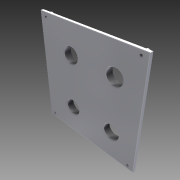
# Autodesk Inventor part: SinglePlane3
Saved by Autodesk Inventor 2015 (Build 190159000, 159)
## iProperties
Created: 2015-03-20
Part Number: SinglePlane3
Material: Aluminum 6061
Document SubType Name: Modeling
Designer: Akovo_000
Density: 2.7 g/cm^3
Appearance: Aluminum - Flat
Mass: 35.5834 g
Surface Area: 130.658 cm^2
Volume: 13.1791 cm^3
Author: Akovo_000
Autodesk Inventor part; units mm, degrees
ref_plane "YZ Plane" through (0, 0, 0) normal (1, 0, 0) x (0, 1, 0)
ref_plane "XZ Plane" through (0, 0, 0) normal (0, 1, 0) x (-1, 0, 0)
ref_plane "XY Plane" through (0, 0, 0) normal (0, 0, 1) x (1, 0, 0)
ref_plane "Main Work Pane" through (0, 2.75, 7) normal (0, 1, 0) x (-1, 0, 0)
sketch "Panel" plane through (0, 2.75, 7) normal (0, 1, 0) x (-1, 0, 0)
  circle A0 centre (8.8252, 26.2409) radius 5.8
  circle A1 centre (8.8252, -12.7591) radius 5.8
  circle A2 centre (42.6252, -12.7591) radius 5.8
  circle A3 centre (42.6252, 26.2409) radius 5.8
  line L0 (42.6252, -12.7591) -> (42.6252, -12.7591)
  line L1 (60.6252, 44.2409) -> (24.6252, 44.2409)
  line L2 (24.6252, 44.2409) -> (24.6252, 8.2409)
  line L3 (24.6252, 8.2409) -> (60.6252, 8.2409)
  line L4 (60.6252, 8.2409) -> (60.6252, 44.2409)
  line L5 (60.6252, 44.2409) -> (24.6252, 8.2409) construction
  line L6 (24.6252, 44.2409) -> (60.6252, 8.2409) construction
  line L7 (60.6252, 5.2409) -> (24.6252, 5.2409)
  line L8 (24.6252, 5.2409) -> (24.6252, -30.7591)
  line L9 (24.6252, -30.7591) -> (60.6252, -30.7591)
  line L10 (60.6252, -30.7591) -> (60.6252, 5.2409)
  line L11 (60.6252, 5.2409) -> (24.6252, -30.7591) construction
  line L12 (24.6252, 5.2409) -> (60.6252, -30.7591) construction
  line L13 (21.6252, 39.0409) -> (-3.9748, 39.0409)
  line L14 (-3.9748, 39.0409) -> (-3.9748, 13.4409)
  line L15 (-3.9748, 13.4409) -> (21.6252, 13.4409)
  line L16 (21.6252, 13.4409) -> (21.6252, 39.0409)
  line L17 (21.6252, 39.0409) -> (-3.9748, 13.4409) construction
  line L18 (-3.9748, 39.0409) -> (21.6252, 13.4409) construction
  line L19 (21.6252, 0.0409) -> (-3.9748, 0.0409)
  line L20 (-3.9748, 0.0409) -> (-3.9748, -25.5591)
  line L21 (-3.9748, -25.5591) -> (21.6252, -25.5591)
  line L22 (21.6252, -25.5591) -> (21.6252, 0.0409)
  line L23 (21.6252, 0.0409) -> (-3.9748, -25.5591) construction
  line L24 (-3.9748, 0.0409) -> (21.6252, -25.5591) construction
  line L25 (60.6252, -30.7591) -> (60.6252, 44.2409)
  line L26 (60.6252, 44.2409) -> (-3.9748, 44.2409)
  line L27 (-3.9748, 44.2409) -> (-3.9748, -30.7591)
  line L28 (-3.9748, -30.7591) -> (60.6252, -30.7591)
  line L29 (68.6252, -33.7591) -> (-9.9748, -33.7591)
  line L30 (-9.9748, -33.7591) -> (-9.9748, 47.2409)
  line L31 (-9.9748, 47.2409) -> (68.6252, 47.2409)
  line L32 (68.6252, 47.2409) -> (68.6252, -33.7591)
  line L33 (42.6252, 20.4409) -> (42.6252, -6.9591)
  line L34 (36.8252, 26.2409) -> (14.6252, 26.2409)
  line L35 (8.8252, 20.4409) -> (8.8252, -6.9591)
  line L36 (14.6252, -12.7591) -> (36.8252, -12.7591)
  dimension "d337" = 11.6
  dimension "d490" = 36
  dimension "d491" = 36
  dimension "d494" = 3
  dimension "d495" = 25.6
  dimension "d496" = 25.6
  dimension "d497" = 3
  dimension "d498" = 0
  dimension "d499" = 8
  dimension "d500" = 6
  dimension "d501" = 3
  dimension "d502" = 3
  dimension "d564" = 81
  dimension "d565" = 78.6
  constraints: 74 end point, 12 parallel, 9 perpendicular, 8 midpoint, 8 point on circle, 6 equal length, 6 line through centre, 5 horizontal, 4 centre point, 3 equal radius, 2 vertical
  measures "d337" diameter of A2
  measures "d490" distance of L3.end L2.end
  measures "d491" distance of L2.end L1.end
  measures "d494" distance between parallel lines of L7 L3
  measures "d495" distance of L15.end L14.end
  measures "d496" distance of L14.end L13.end
  measures "d497" distance between parallel lines of L22 L8
  measures "d498" distance between parallel lines of L27 L14
  measures "d499" distance between parallel lines of L32 L25
  measures "d500" distance between parallel lines of L30 L27
  measures "d501" distance between parallel lines of L31 L1
  measures "d502" distance between parallel lines of L29 L28
  measures "d564" distance between parallel lines of L29 L31
  measures "d565" distance between parallel lines of L32 L30
extrude "Panel3D" add sketch "Panel" along normal blind 2 contours L34 L16 L15 L35 A0 | A0 L35 L15 L14 L13 L16 L34 | L34 L2 L3 L33 L7 L8 L36 L22 L19 L35 L15 L16 | L16 L13 L27 L26 L2 L34 | L35 L19 L27 L15 | L34 A3 L33 L3 L2 | L2 L1 L4 L3 L33 A3 L34 | L35 A1 L36 L22 L21 L20 L19 | L19 L22 L36 A1 L35 | L3 L25 L7 L33 | L21 L22 L36 L8 L28 L27 | L33 A2 L36 L8 L7 | L7 L10 L9 L8 L36 A2 L33 | L29 L30 L31 L32
sketch "BoardSuport" plane through (0, 2.75, 7) normal (0, -1, 0) x (1, 0, 0)
  line L0 (-58.1252, 41.7409) -> (-27.1252, 41.7409)
  line L1 (-27.1252, 41.7409) -> (-27.1252, 10.7409)
  line L2 (-27.1252, 10.7409) -> (-58.1252, 10.7409)
  line L3 (-58.1252, 10.7409) -> (-58.1252, 41.7409)
  circle A0 centre (-42.6252, 26.2409) radius 5.8 projected
  line L4 (-58.1252, 41.7409) -> (-27.1252, 10.7409) construction
  line L5 (-27.1252, 41.7409) -> (-58.1252, 10.7409) construction
  line L6 (-58.1252, 2.7409) -> (-27.1252, 2.7409)
  line L7 (-27.1252, 2.7409) -> (-27.1252, -28.2591)
  line L8 (-27.1252, -28.2591) -> (-58.1252, -28.2591)
  line L9 (-58.1252, -28.2591) -> (-58.1252, 2.7409)
  circle A1 centre (-42.6252, -12.7591) radius 5.8 projected
  line L10 (-58.1252, 2.7409) -> (-27.1252, -28.2591) construction
  line L11 (-27.1252, 2.7409) -> (-58.1252, -28.2591) construction
  line L12 (-20.0752, 37.4909) -> (2.4248, 37.4909)
  line L13 (2.4248, 37.4909) -> (2.4248, 14.9909)
  line L14 (2.4248, 14.9909) -> (-20.0752, 14.9909)
  line L15 (-20.0752, 14.9909) -> (-20.0752, 37.4909)
  circle A2 centre (-8.8252, 26.2409) radius 5.8 projected
  line L16 (-20.0752, 37.4909) -> (2.4248, 14.9909) construction
  line L17 (2.4248, 37.4909) -> (-20.0752, 14.9909) construction
  line L18 (-20.0752, -1.5091) -> (2.4248, -1.5091)
  line L19 (2.4248, -1.5091) -> (2.4248, -24.0091)
  line L20 (2.4248, -24.0091) -> (-20.0752, -24.0091)
  line L21 (-20.0752, -24.0091) -> (-20.0752, -1.5091)
  circle A3 centre (-8.8252, -12.7591) radius 5.8 projected
  line L22 (-20.0752, -1.5091) -> (2.4248, -24.0091) construction
  line L23 (2.4248, -1.5091) -> (-20.0752, -24.0091) construction
  line L24 (-60.2252, 4.8409) -> (-56.0252, 4.8409)
  line L25 (-56.0252, 4.8409) -> (-56.0252, 0.6409)
  line L26 (-56.0252, 0.6409) -> (-60.2252, 0.6409)
  line L27 (-60.2252, 0.6409) -> (-60.2252, 4.8409)
  line L28 (-60.2252, 4.8409) -> (-56.0252, 0.6409) construction
  line L29 (-56.0252, 4.8409) -> (-60.2252, 0.6409) construction
  line L30 (-60.2252, 12.8409) -> (-56.0252, 12.8409)
  line L31 (-56.0252, 12.8409) -> (-56.0252, 8.6409)
  line L32 (-56.0252, 8.6409) -> (-60.2252, 8.6409)
  line L33 (-60.2252, 8.6409) -> (-60.2252, 12.8409)
  line L34 (-60.2252, 12.8409) -> (-56.0252, 8.6409) construction
  line L35 (-56.0252, 12.8409) -> (-60.2252, 8.6409) construction
  line L36 (-29.2252, 12.8409) -> (-25.0252, 12.8409)
  line L37 (-25.0252, 12.8409) -> (-25.0252, 8.6409)
  line L38 (-25.0252, 8.6409) -> (-29.2252, 8.6409)
  line L39 (-29.2252, 8.6409) -> (-29.2252, 12.8409)
  line L40 (-29.2252, 12.8409) -> (-25.0252, 8.6409) construction
  line L41 (-25.0252, 12.8409) -> (-29.2252, 8.6409) construction
  line L42 (-29.2252, 43.8409) -> (-25.0252, 43.8409)
  line L43 (-25.0252, 43.8409) -> (-25.0252, 39.6409)
  line L44 (-25.0252, 39.6409) -> (-29.2252, 39.6409)
  line L45 (-29.2252, 39.6409) -> (-29.2252, 43.8409)
  line L46 (-29.2252, 43.8409) -> (-25.0252, 39.6409) construction
  line L47 (-25.0252, 43.8409) -> (-29.2252, 39.6409) construction
  line L48 (-60.2252, 43.8409) -> (-56.0252, 43.8409)
  line L49 (-56.0252, 43.8409) -> (-56.0252, 39.6409)
  line L50 (-56.0252, 39.6409) -> (-60.2252, 39.6409)
  line L51 (-60.2252, 39.6409) -> (-60.2252, 43.8409)
  line L52 (-60.2252, 43.8409) -> (-56.0252, 39.6409) construction
  line L53 (-56.0252, 43.8409) -> (-60.2252, 39.6409) construction
  line L54 (-29.2252, 4.8409) -> (-25.0252, 4.8409)
  line L55 (-25.0252, 4.8409) -> (-25.0252, 0.6409)
  line L56 (-25.0252, 0.6409) -> (-29.2252, 0.6409)
  line L57 (-29.2252, 0.6409) -> (-29.2252, 4.8409)
  line L58 (-29.2252, 4.8409) -> (-25.0252, 0.6409) construction
  line L59 (-25.0252, 4.8409) -> (-29.2252, 0.6409) construction
  line L60 (-29.2252, -26.1591) -> (-25.0252, -26.1591)
  line L61 (-25.0252, -26.1591) -> (-25.0252, -30.3591)
  line L62 (-25.0252, -30.3591) -> (-29.2252, -30.3591)
  line L63 (-29.2252, -30.3591) -> (-29.2252, -26.1591)
  line L64 (-29.2252, -26.1591) -> (-25.0252, -30.3591) construction
  line L65 (-25.0252, -26.1591) -> (-29.2252, -30.3591) construction
  line L66 (-60.2252, -26.1591) -> (-56.0252, -26.1591)
  line L67 (-56.0252, -26.1591) -> (-56.0252, -30.3591)
  line L68 (-56.0252, -30.3591) -> (-60.2252, -30.3591)
  line L69 (-60.2252, -30.3591) -> (-60.2252, -26.1591)
  line L70 (-60.2252, -26.1591) -> (-56.0252, -30.3591) construction
  line L71 (-56.0252, -26.1591) -> (-60.2252, -30.3591) construction
  line L72 (-21.5752, -22.5091) -> (-18.5752, -22.5091)
  line L73 (-18.5752, -22.5091) -> (-18.5752, -25.5091)
  line L74 (-18.5752, -25.5091) -> (-21.5752, -25.5091)
  line L75 (-21.5752, -25.5091) -> (-21.5752, -22.5091)
  line L76 (-21.5752, -22.5091) -> (-18.5752, -25.5091) construction
  line L77 (-18.5752, -22.5091) -> (-21.5752, -25.5091) construction
  line L78 (0.9248, -22.5091) -> (3.9248, -22.5091)
  line L79 (3.9248, -22.5091) -> (3.9248, -25.5091)
  line L80 (3.9248, -25.5091) -> (0.9248, -25.5091)
  line L81 (0.9248, -25.5091) -> (0.9248, -22.5091)
  line L82 (0.9248, -22.5091) -> (3.9248, -25.5091) construction
  line L83 (3.9248, -22.5091) -> (0.9248, -25.5091) construction
  line L84 (0.9248, -0.0091) -> (3.9248, -0.0091)
  line L85 (3.9248, -0.0091) -> (3.9248, -3.0091)
  line L86 (3.9248, -3.0091) -> (0.9248, -3.0091)
  line L87 (0.9248, -3.0091) -> (0.9248, -0.0091)
  line L88 (0.9248, -0.0091) -> (3.9248, -3.0091) construction
  line L89 (3.9248, -0.0091) -> (0.9248, -3.0091) construction
  line L90 (-21.5752, -0.0091) -> (-18.5752, -0.0091)
  line L91 (-18.5752, -0.0091) -> (-18.5752, -3.0091)
  line L92 (-18.5752, -3.0091) -> (-21.5752, -3.0091)
  line L93 (-21.5752, -3.0091) -> (-21.5752, -0.0091)
  line L94 (-21.5752, -0.0091) -> (-18.5752, -3.0091) construction
  line L95 (-18.5752, -0.0091) -> (-21.5752, -3.0091) construction
  line L96 (-21.5752, 13.4909) -> (-18.5752, 13.4909)
  line L97 (-18.5752, 13.4909) -> (-18.5752, 16.4909)
  line L98 (-18.5752, 16.4909) -> (-21.5752, 16.4909)
  line L99 (-21.5752, 16.4909) -> (-21.5752, 13.4909)
  line L100 (-21.5752, 13.4909) -> (-18.5752, 16.4909) construction
  line L101 (-18.5752, 13.4909) -> (-21.5752, 16.4909) construction
  line L102 (3.9248, 13.4909) -> (0.9248, 13.4909)
  line L103 (0.9248, 13.4909) -> (0.9248, 16.4909)
  line L104 (0.9248, 16.4909) -> (3.9248, 16.4909)
  line L105 (3.9248, 16.4909) -> (3.9248, 13.4909)
  line L106 (3.9248, 13.4909) -> (0.9248, 16.4909) construction
  line L107 (0.9248, 13.4909) -> (3.9248, 16.4909) construction
  line L108 (3.9248, 38.9909) -> (0.9248, 38.9909)
  line L109 (0.9248, 38.9909) -> (0.9248, 35.9909)
  line L110 (0.9248, 35.9909) -> (3.9248, 35.9909)
  line L111 (3.9248, 35.9909) -> (3.9248, 38.9909)
  line L112 (3.9248, 38.9909) -> (0.9248, 35.9909) construction
  line L113 (0.9248, 38.9909) -> (3.9248, 35.9909) construction
  line L114 (-21.5752, 38.9909) -> (-18.5752, 38.9909)
  line L115 (-18.5752, 38.9909) -> (-18.5752, 35.9909)
  line L116 (-18.5752, 35.9909) -> (-21.5752, 35.9909)
  line L117 (-21.5752, 35.9909) -> (-21.5752, 38.9909)
  line L118 (-21.5752, 38.9909) -> (-18.5752, 35.9909) construction
  line L119 (-18.5752, 38.9909) -> (-21.5752, 35.9909) construction
  arc A4 (-58.1252, 39.6409) -> (-56.0252, 41.7409) centre (-58.1252, 41.7409) ccw
  arc A5 (-29.2252, 41.7409) -> (-27.1252, 39.6409) centre (-27.1252, 41.7409) ccw
  arc A6 (-27.1252, 12.8409) -> (-29.2252, 10.7409) centre (-27.1252, 10.7409) ccw
  arc A7 (-56.0252, 10.7409) -> (-58.1252, 12.8409) centre (-58.1252, 10.7409) ccw
  arc A8 (-58.1252, 0.6409) -> (-56.0252, 2.7409) centre (-58.1252, 2.7409) ccw
  arc A9 (-56.0252, -28.2591) -> (-58.1252, -26.1591) centre (-58.1252, -28.2591) ccw
  arc A10 (-27.1252, -26.1591) -> (-29.2252, -28.2591) centre (-27.1252, -28.2591) ccw
  arc A11 (-18.5752, -24.0091) -> (-20.0752, -22.5091) centre (-20.0752, -24.0091) ccw
  arc A12 (2.4248, -22.5091) -> (0.9248, -24.0091) centre (2.4248, -24.0091) ccw
  arc A13 (0.9248, -1.5091) -> (2.4248, -3.0091) centre (2.4248, -1.5091) ccw
  arc A14 (-20.0752, -3.0091) -> (-18.5752, -1.5091) centre (-20.0752, -1.5091) ccw
  arc A15 (-29.2252, 2.7409) -> (-27.1252, 0.6409) centre (-27.1252, 2.7409) ccw
  arc A16 (-20.0752, 35.9909) -> (-18.5752, 37.4909) centre (-20.0752, 37.4909) ccw
  arc A17 (-18.5752, 14.9909) -> (-20.0752, 16.4909) centre (-20.0752, 14.9909) ccw
  arc A18 (2.4248, 16.4909) -> (0.9248, 14.9909) centre (2.4248, 14.9909) ccw
  arc A19 (0.9248, 37.4909) -> (2.4248, 35.9909) centre (2.4248, 37.4909) ccw
  circle A20 centre (-58.1252, 41.7409) radius 0.8
  circle A21 centre (-58.1252, 10.7409) radius 0.8
  circle A22 centre (-27.1252, 10.7409) radius 0.8
  circle A23 centre (-27.1252, 41.7409) radius 0.8
  circle A24 centre (-58.1252, 2.7409) radius 0.8
  circle A25 centre (-58.1252, -28.2591) radius 0.8
  circle A26 centre (-27.1252, -28.2591) radius 0.8
  circle A27 centre (-27.1252, 2.7409) radius 0.8
  circle A28 centre (-20.0752, -1.5091) radius 0.8
  circle A29 centre (-20.0752, -24.0091) radius 0.8
  circle A30 centre (2.4248, -24.0091) radius 0.8
  circle A31 centre (2.4248, -1.5091) radius 0.8
  circle A32 centre (2.4248, 14.9909) radius 0.8
  circle A33 centre (-20.0752, 14.9909) radius 0.8
  circle A34 centre (2.4248, 37.4909) radius 0.8
  circle A35 centre (-20.0752, 37.4909) radius 0.8
  dimension "d540" = 31
  dimension "d541" = 31
  dimension "d542" = 22.5
  dimension "d543" = 22.5
  dimension "d545" = 4.2
  dimension "d546" = 3
  dimension "d547" = 1.6
  dimension "d548" = 1.6
  constraints: 240 end point, 76 midpoint, 40 parallel, 32 centre point, 32 point on circle, 20 horizontal, 20 perpendicular, 18 point on line, 16 equal length, 16 tangent, 14 coincident, 14 equal radius
  measures "d540" distance of L1.end L2.end
  measures "d541" distance of L0.end L1.end
  measures "d542" distance of L13.end L14.end
  measures "d543" distance of L12.end L13.end
  measures "d545" distance between parallel lines of L24 L26
  measures "d546" distance between parallel lines of L80 L78
  measures "d547" diameter of A25
  measures "d548" diameter of A30
extrude "BoardSupport3D" [suppressed]
sketch "PlasticMount Hole Position" plane through (0, 2.75, 7) normal (0, -1, 0) x (1, 0, 0)
  line L0 (9.9748, 47.2409) -> (-68.6252, 47.2409)
  line L1 (-68.6252, 47.2409) -> (-68.6252, -33.7591)
  line L2 (-68.6252, -33.7591) -> (9.9748, -33.7591)
  line L3 (9.9748, -33.7591) -> (9.9748, 47.2409)
  line L4 (-68.6252, -33.7591) -> (-64.1252, -33.7591)
  line L5 (-64.1252, -33.7591) -> (-64.1252, -30.7591)
  line L6 (-64.1252, -30.7591) -> (-68.6252, -30.7591)
  line L7 (-68.6252, -30.7591) -> (-68.6252, -33.7591)
  line L8 (-68.6252, 47.2409) -> (-64.1252, 47.2409)
  line L9 (-64.1252, 47.2409) -> (-64.1252, 44.2409)
  line L10 (-64.1252, 44.2409) -> (-68.6252, 44.2409)
  line L11 (-68.6252, 44.2409) -> (-68.6252, 47.2409)
  line L12 (9.9748, 47.2409) -> (5.4748, 47.2409)
  line L13 (5.4748, 47.2409) -> (5.4748, 44.2409)
  line L14 (5.4748, 44.2409) -> (9.9748, 44.2409)
  line L15 (9.9748, 44.2409) -> (9.9748, 47.2409)
  line L16 (9.9748, -33.7591) -> (5.4748, -33.7591)
  line L17 (5.4748, -33.7591) -> (5.4748, -30.7591)
  line L18 (5.4748, -30.7591) -> (9.9748, -30.7591)
  line L19 (9.9748, -30.7591) -> (9.9748, -33.7591)
  point P0 (0, -7)
  dimension "d554" = 4.5
  dimension "d555" = 3
  constraints: 40 end point, 10 parallel, 5 equal length, 5 horizontal, 5 perpendicular, 2 point on line
  measures "d554" distance between parallel lines of L19 L17
  measures "d555" distance between parallel lines of L18 L16
hole "PlasticMountHoles" at (5.4748, 2.75, 51.2409) at (-64.1252, 2.75, -23.7591) at (5.4748, 2.75, -23.7591) at (-64.1252, 2.75, 51.2409) direction (0, 1, 0) diameter 1.6 depth 4 tip angle 118
sketch "Lens and screwcover" plane through (0, 4.75, 7) normal (0, 1, 0) x (1, 0, 0)
  circle A0 centre (-42.6252, -26.2409) radius 5.8 projected
  circle A1 centre (-42.6252, -26.2409) radius 5.8
  circle A2 centre (-8.8252, -26.2409) radius 5.8 projected
  circle A3 centre (-8.8252, -26.2409) radius 5.8
  circle A4 centre (-8.8252, 12.7591) radius 5.8 projected
  circle A5 centre (-8.8252, 12.7591) radius 5.8
  circle A6 centre (-42.6252, 12.7591) radius 5.8 projected
  circle A7 centre (-42.6252, 12.7591) radius 5.8
  circle A8 centre (-42.6252, -26.2409) radius 8.3
  circle A9 centre (-8.8252, -26.2409) radius 8.3
  circle A10 centre (-8.8252, 12.7591) radius 8.3
  circle A11 centre (-42.6252, 12.7591) radius 8.3
  circle A12 centre (5.4748, -44.2409) radius 0.8 projected
  circle A13 centre (5.4748, -44.2409) radius 1.8
  circle A14 centre (3.9748, 30.8158) radius 1.8
  circle A15 centre (-64.1252, 30.7591) radius 0.8 projected
  circle A16 centre (-64.1252, 30.7591) radius 1.8
  circle A17 centre (-64.1252, -44.2409) radius 0.8 projected
  circle A18 centre (-64.1252, -44.2409) radius 1.8
  point P0 (0, 7)
  dimension "d551" = 2.5
  dimension "d563" = 1
  constraints: 12 centre point, 11 coincident, 6 equal radius
  measures "d551" radial gap between concentric circles of A8 A0
  measures "d563" radial gap between concentric circles of A18 A17
extrude "Extrusion15" add sketch "Lens and screwcover" along normal blind 3 contours A8 | A9 | A10 | A11 | A12 | A13 | A14 | A15 | A16 | A17 | A18
thread "Lensthread" size "M12x0.5" class "6H" standard "ANSI Metric M Profile" full length
thread "LensThread2" size "M12x0.5" class "6H" standard "ANSI Metric M Profile" full length
thread "LensThread3" size "M12x0.5" class "6H" standard "ANSI Metric M Profile" full length
thread "LensThread4" size "M12x0.5" class "6H" standard "ANSI Metric M Profile" full length
thread "MountThread1" size "M2x0.4" class "6H" standard "ANSI Metric M Profile" full length
thread "Thread18" size "M2x0.4" class "6H" standard "ANSI Metric M Profile" full length
thread "Thread19" size "M2x0.4" class "6H" standard "ANSI Metric M Profile" full length
thread "Thread20" size "M2x0.4" class "6H" standard "ANSI Metric M Profile" full length
body "Solid3"
